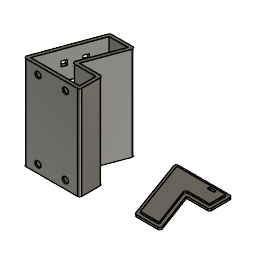
case_only (Autodesk Fusion 360 design; units mm, degrees)
part number: 2026-03-11-12-51-07-176
Autodesk Fusion 360 part; units mm, degrees
sketch "Sketch1" plane through (0, 0, 0) normal (0, 0, 1) x (1, 0, 0)
  line L0 (-379.8243, -255.6139) -> (-354.1728, -185.137)
  line L1 (-379.8243, -255.6139) -> (-454.8243, -255.6139) construction
  line L2 (-379.8243, -255.6139) -> (-319.8243, -255.6139)
  line L3 (-319.8243, -255.6139) -> (-319.8243, -235.6139)
  line L4 (-319.8243, -235.6139) -> (-349.8243, -235.6139)
  line L5 (-349.8243, -235.6139) -> (-331, -185)
  line L6 (-331, -185) -> (-354.1728, -185.137)
  line L7 (-325.2319, -180.9658) -> (-356.9796, -181.1535)
  line L8 (-385.5369, -259.6139) -> (-356.9796, -181.1535)
  line L9 (-385.5369, -259.6139) -> (-315.8243, -259.6139)
  line L10 (-315.8243, -259.6139) -> (-315.8243, -231.6139)
  line L11 (-315.8243, -231.6139) -> (-344.0689, -231.6139)
  line L12 (-344.0689, -231.6139) -> (-325.2319, -180.9658)
  dimension "d11" = 110
  dimension "d12" = 75
  dimension "d13" = 60
  dimension "d14" = 20
  dimension "d15" = 30
  dimension "d16" = -4
  constraint horizontal L1
  constraint parallel L1 L2
  constraint perpendicular L2 L3
  constraint perpendicular L3 L4
  measures "d11" angle of L0 L1
  measures "d12" distance of L0.start L0.end
  measures "d13" distance of L0.start L2.end
  measures "d14" distance of L2.end L3.end
  measures "d15" distance of L3.end L4.end
extrude "Extrude1" add sketch "Sketch1" along normal blind 115 makes body 1
extrude "Extrude2" add sketch "Sketch1" along normal blind 2.5 contours L0 L2 L3 L4 L5 L6 bodies 1
fillet "Fillet1" radius 2.5 1 edges at (-325.2319, -180.9658, 57.5) on bodies 1
fillet "Fillet2" radius 2.5 1 edges at (-385.5369, -259.6139, 57.5) on bodies 1
fillet "Fillet3" radius 2.5 1 edges at (-356.9796, -181.1535, 57.5) on bodies 1
fillet "Fillet4" radius 2.5 1 edges at (-349.8243, -235.6139, 58.75) on bodies 1
fillet "Fillet5" radius 2.5 1 edges at (-315.8243, -259.6139, 57.5) on bodies 1
fillet "Fillet6" radius 2.5 1 edges at (-315.8243, -231.6139, 57.5) on bodies 1
sketch "Sketch2" plane through (0, 0, 115) normal (0, 0, 1) x (-1, 0, 0)
  arc A0 (315.8243, 234.1139) -> (318.3243, 231.6139) centre (318.3243, 234.1139) ccw
  line L0 (318.3243, 231.6139) -> (344.0689, 231.6139)
  line L1 (344.0689, 231.6139) -> (326.4938, 184.3587)
  arc A1 (326.4938, 184.3587) -> (328.8518, 180.9872) centre (328.837, 183.4872) ccw
  line L2 (328.8518, 180.9872) -> (355.2401, 181.1432)
  arc A2 (355.2401, 181.1432) -> (357.5746, 182.7881) centre (355.2253, 183.6432) ccw
  line L3 (357.5746, 182.7881) -> (384.3157, 256.2589)
  arc A3 (384.3157, 256.2589) -> (381.9665, 259.6139) centre (381.9665, 257.1139) ccw
  line L4 (381.9665, 259.6139) -> (318.3243, 259.6139)
  arc A4 (318.3243, 259.6139) -> (315.8243, 257.1139) centre (318.3243, 257.1139) ccw
  line L5 (315.8243, 257.1139) -> (315.8243, 234.1139)
  arc A5 (348.5704, 232.2425) -> (346.2272, 235.6139) centre (346.2272, 233.1139) ccw
  line L6 (346.2272, 235.6139) -> (319.8243, 235.6139)
  line L7 (319.8243, 235.6139) -> (319.8243, 255.6139)
  line L8 (319.8243, 255.6139) -> (379.8243, 255.6139)
  line L9 (379.8243, 255.6139) -> (354.1728, 185.137)
  line L10 (354.1728, 185.137) -> (331, 185)
  line L11 (331, 185) -> (348.5704, 232.2425)
extrude "Extrude3" add sketch "Sketch2" along normal blind 2.5 separate body makes body 2
extrude "Extrude4" add 1 faces at (-360.8558, -224.3311, 2.5) along direction (0, 0, 1) blind 4.5 separate body on bodies 1 makes body 3
move_face "MoveFace1" by (70, 0, 0) 1 faces at (-360.8558, -224.3311, 7) on bodies 3
move_body "Move1" bodies 3 to x (1, 0, 0) y (0, 1, 0) z (0, 0, 1) at (80, 0, 0)
move_body "Move2" bodies 2 to x (1, 0, 0) y (0, 1, 0) z (0, 0, 1) at (80, 0, 0)
move_body "Move3" bodies 2 to x (1, 0, 0) y (0, 1, 0) z (0, 0, 1) at (0, 0, -112.4)
move_body "Move4" bodies 2 to x (1, 0, 0) y (0, 1, 0) z (0, 0, 1) at (0, 0, -0.1)
move_body "Move5" bodies 2 to x (1, 0, 0) y (0, 1, 0) z (0, 0, 1) at (0, 0, 2)
combine "Combine1" operation add target body 2 tool bodies 3
sketch "Sketch3" plane through (-256.9993, 93.5401, 0) normal (-0.939693, 0.34202, 0) x (-0.34202, -0.939693, 0)
  line L0 (294.0624, 115) -> (294.0624, 0)
  line L1 (294.0624, 0) -> (372.2483, 0)
  line L2 (372.2483, 0) -> (372.2483, 115)
  line L3 (372.2483, 115) -> (294.0624, 115)
  line L4 (308.1554, 81) -> (358.1554, 81)
  line L5 (358.1554, 81) -> (358.1554, 15)
  line L6 (358.1554, 15) -> (308.1554, 15)
  line L7 (308.1554, 15) -> (308.1554, 81)
  line L8 (375.8187, 0) -> (292.3228, 0)
  dimension "d37" = 50
  dimension "d38" = 66
  dimension "d39" = 14.093
  dimension "d40" = 15
  constraint horizontal L4
  constraint vertical L5
  constraint horizontal L6
  constraint vertical L7
  measures "d37" distance of L4.start L4.end
  measures "d38" distance of L4.start L6.end
  measures "d39" distance of L0 L7
  measures "d40" distance of L6 L8
extrude "Extrude5" cut sketch "Sketch3" against normal blind 10 draft -10 contours L4 L5 L6 L7 bodies 1
sketch "Sketch4" plane through (0, 0, 7) normal (0, 0, 1) x (-1, 0, 0)
  line L0 (235.8243, 257.1139) -> (235.8243, 234.1139)
  arc A0 (235.8243, 234.1139) -> (238.3243, 231.6139) centre (238.3243, 234.1139) ccw
  line L1 (238.3243, 231.6139) -> (264.0689, 231.6139)
  line L2 (264.0689, 231.6139) -> (246.4938, 184.3587)
  arc A1 (246.4938, 184.3587) -> (248.8518, 180.9872) centre (248.837, 183.4872) ccw
  line L3 (248.8518, 180.9872) -> (275.2401, 181.1432)
  arc A2 (275.2401, 181.1432) -> (277.5746, 182.7881) centre (275.2253, 183.6432) ccw
  line L4 (277.5746, 182.7881) -> (304.3157, 256.2589)
  arc A3 (304.3157, 256.2589) -> (301.9665, 259.6139) centre (301.9665, 257.1139) ccw
  line L5 (301.9665, 259.6139) -> (238.3243, 259.6139)
  arc A4 (238.3243, 259.6139) -> (235.8243, 257.1139) centre (238.3243, 257.1139) ccw
move_body "Move6" bodies 2 to x (1, 0, 0) y (0, -1, 0) z (0, 0, -1) at (0, -511.2279, 0)
move_body "Move7" bodies 2 to x (1, 0, 0) y (0, 1, 0) z (0, 0, 1) at (7.7237, 91.7881, 0)
sketch "Sketch5" plane through (0, -259.6139, 0) normal (0, -1, 0) x (1, 0, 0)
  line L0 (-318.3243, 0) -> (-318.3243, 115)
  line L1 (-318.3243, 115) -> (-381.9665, 115)
  line L2 (-381.9665, 115) -> (-381.9665, 0)
  line L3 (-381.9665, 0) -> (-318.3243, 0)
  circle A0 centre (-366.9665, 105) radius 3.75
  circle A1 centre (-333.3243, 105) radius 3.75
  circle A2 centre (-333.3243, 10) radius 3.75
  circle A3 centre (-366.9665, 10) radius 3.75
  dimension "d44" = 7.5
  dimension "d45" = 10
  dimension "d46" = 15
  dimension "d47" = 7.5
  dimension "d48" = 10
  dimension "d49" = 15
  dimension "d50" = 7.5
  dimension "d51" = 15
  dimension "d52" = 10
  dimension "d53" = 7.5
  dimension "d54" = 10
  dimension "d55" = 15
  measures "d44" diameter of A0
  measures "d45" distance of L1 A0.centre
  measures "d46" distance of L2 A0.centre
  measures "d47" diameter of A1
  measures "d48" distance of L1 A1.centre
  measures "d49" distance of L0 A1.centre
  measures "d50" diameter of A2
  measures "d51" distance of L0 A2.centre
  measures "d52" distance of L3 A2.centre
  measures "d53" diameter of A3
  measures "d54" distance of L3 A3.centre
  measures "d55" distance of L2 A3.centre
extrude "Extrude6" cut sketch "Sketch5" against normal blind 1.5 draft -10 contours A0 | A1 | A2 | A3 bodies 1
sketch "Sketch6" plane through (0, 0, -7) normal (0, 0, -1) x (1, 0, 0)
  line L0 (-228.1005, 162.3258) -> (-228.1005, 185.3258)
  arc A0 (-228.1005, 185.3258) -> (-230.6005, 187.8258) centre (-230.6005, 185.3258) ccw
  line L1 (-230.6005, 187.8258) -> (-256.3452, 187.8258)
  line L2 (-256.3452, 187.8258) -> (-238.7701, 235.0811)
  arc A1 (-238.7701, 235.0811) -> (-241.128, 238.4526) centre (-241.1133, 235.9526) ccw
  line L3 (-241.128, 238.4526) -> (-267.5164, 238.2965)
  arc A2 (-267.5164, 238.2965) -> (-269.8508, 236.6516) centre (-267.5016, 235.7966) ccw
  line L4 (-269.8508, 236.6516) -> (-296.592, 163.1809)
  arc A3 (-296.592, 163.1809) -> (-294.2428, 159.8258) centre (-294.2428, 162.3258) ccw
  line L5 (-294.2428, 159.8258) -> (-230.6005, 159.8258)
  arc A4 (-230.6005, 159.8258) -> (-228.1005, 162.3258) centre (-230.6005, 162.3258) ccw
  line L6 (-249, 168.7758) -> (-242.6, 168.7758)
  line L7 (-241.6, 167.7758) -> (-241.6, 167.1758)
  line L8 (-242.6, 166.1758) -> (-249, 166.1758)
  line L9 (-250, 167.1758) -> (-250, 167.7758)
  arc A5 (-249, 168.7758) -> (-250, 167.7758) centre (-249, 167.7758) ccw
  arc A6 (-250, 167.1758) -> (-249, 166.1758) centre (-249, 167.1758) ccw
  arc A7 (-241.6, 167.7758) -> (-242.6, 168.7758) centre (-242.6, 167.7758) ccw
  arc A8 (-242.6, 166.1758) -> (-241.6, 167.1758) centre (-242.6, 167.1758) ccw
  point P0 (-250, 168.7758)
  point P1 (-241.6, 168.7758)
  point P2 (-250, 166.1758)
  dimension "d58" = 8.4
  dimension "d59" = 2.6
  dimension "d60" = 1
  dimension "d61" = 6.35
  constraint horizontal L6
  constraint vertical L7
  constraint horizontal L8
  constraint vertical L9
  constraint coincident P0 L6
  constraint coincident P0 L9
  constraint tangent L6 A5
  constraint tangent L9 A5
  constraint coincident P2 L8
  constraint coincident P2 L9
  constraint tangent L8 A6
  constraint tangent L9 A6
  constraint equal A5 A6
  constraint coincident P1 L6
  constraint coincident P1 L7
  constraint tangent L6 A7
  constraint tangent L7 A7
  constraint equal A5 A7
  constraint tangent L7 A8
  constraint tangent L8 A8
  constraint equal A5 A8
  measures "d58" distance of P0 P1
  measures "d59" distance of P0 P2
  measures "d60" radius of A5
  measures "d61" distance of L5 L8
extrude "Extrude7" cut sketch "Sketch6" against normal blind 5 contours L6 L7 L8 L9 A5 A6 A7 A8 bodies 2
sketch "Sketch7" plane through (-256.9993, 93.5401, 0) normal (-0.939693, 0.34202, 0) x (-0.34202, -0.939693, 0)
  line L0 (358.1554, 81) -> (358.1554, 15)
  line L1 (358.1554, 15) -> (308.1554, 15)
  line L2 (308.1554, 15) -> (308.1554, 81)
  line L3 (308.1554, 81) -> (358.1554, 81)
  line L4 (294.0624, 115) -> (294.0624, 0)
  line L5 (294.0624, 0) -> (372.2483, 0)
  line L6 (372.2483, 0) -> (372.2483, 115)
  line L7 (372.2483, 115) -> (294.0624, 115)
  line L8 (314.0624, 102.5) -> (320.0624, 102.5)
  line L9 (320.0624, 102.5) -> (320.0624, 96.5)
  line L10 (320.0624, 96.5) -> (314.0624, 96.5)
  line L11 (314.0624, 96.5) -> (314.0624, 102.5)
  line L12 (335.0624, 102.5) -> (341.0624, 102.5)
  line L13 (341.0624, 102.5) -> (341.0624, 96.5)
  line L14 (341.0624, 96.5) -> (335.0624, 96.5)
  line L15 (335.0624, 96.5) -> (335.0624, 102.5)
  dimension "d64" = 6
  dimension "d65" = 6
  dimension "d66" = 20
  dimension "d67" = 6
  dimension "d68" = 6
  dimension "d69" = 12.5
  dimension "d70" = 12.5
  dimension "d71" = 15
  constraint horizontal L8
  constraint vertical L9
  constraint horizontal L10
  constraint vertical L11
  constraint horizontal L12
  constraint vertical L13
  constraint horizontal L14
  constraint vertical L15
  measures "d64" distance of L8.start L8.end
  measures "d65" distance of L8.start L10.end
  measures "d66" distance of L4 L11
  measures "d67" distance of L12.start L12.end
  measures "d68" distance of L12.start L14.end
  measures "d69" distance of L7 L8
  measures "d70" distance of L7 L12
  measures "d71" distance of L9 L15
extrude "Extrude8" cut sketch "Sketch7" against normal blind 5 contours L8 L9 L10 L11 | L12 L13 L14 L15 bodies 1
